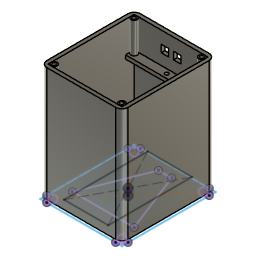
Down_Layer v36 (Autodesk Fusion 360 design; units mm, degrees)
Autodesk Fusion 360 part; units mm, degrees
sketch "Sketch1" plane through (0, 0, 0) normal (0, 0, 1) x (1, 0, 0) in component "Upper Layer"
  line L0 (30, -35) -> (-30, -35)
  line L1 (-30, -35) -> (-30, 35)
  line L2 (-30, 35) -> (30, 35)
  line L3 (30, 35) -> (30, -35)
  line L4 (0, 0) -> (-20, 0) construction
  line L5 (-30, 0) -> (-18, 0) construction
  line L6 (0, -35) -> (0, 35)
  line L7 (-30, -35) -> (0, 0) construction
  line L8 (30, 35) -> (0, 0) construction
  line L9 (-28, 38) -> (28, 38)
  line L10 (33, 33) -> (33, -33)
  line L11 (28, -38) -> (-28, -38)
  line L12 (-33, -33) -> (-33, 33)
  line L13 (-33, 38) -> (33, -38) construction
  line L14 (33, 38) -> (-33, -38) construction
  arc A0 (-33, -33) -> (-28, -38) centre (-28, -33) ccw
  arc A1 (33, 33) -> (28, 38) centre (28, 33) ccw
  arc A2 (28, -38) -> (33, -33) centre (28, -33) ccw
  arc A3 (-28, 38) -> (-33, 33) centre (-28, 33) ccw
  dimension "d1" = 60
  dimension "d2" = 70
  dimension "d27" = 12
  dimension "d33" = 66
  dimension "d34" = 76
  dimension "d110" = 5
  dimension "d111" = 5
  dimension "d112" = 5
  dimension "d113" = 5
  constraint horizontal L0
  constraint perpendicular L0 L1
  constraint parallel L0 L2
  constraint parallel L1 L3
  constraint coincident L4.start L7.end
  constraint horizontal L4
  constraint midpoint L1 L5.start
  constraint perpendicular L1 L5
  constraint midpoint L0 L6.start
  constraint midpoint L2 L6.end
  constraint parallel L7 L8
  constraint horizontal L9
  constraint perpendicular L9 L10
  constraint parallel L9 L11
  constraint parallel L10 L12
  constraint coincident L13 L4.start
  constraint coincident L14 L4.start
  constraint coincident L14.end L11
  constraint coincident L14.end L12
  constraint tangent L11 A0
  constraint tangent L12 A0
  constraint coincident L14.start L10
  constraint coincident L14.start L9
  constraint tangent L10 A1
  constraint tangent L9 A1
  constraint coincident L13.end L10
  constraint coincident L13.end L11
  constraint tangent L10 A2
  constraint tangent L11 A2
  constraint coincident L13.start L9
  constraint coincident L13.start L12
  constraint tangent L9 A3
  constraint tangent L12 A3
  measures "d1" distance of L1.end L2.end
  measures "d2" distance of L0.end L1.end
  measures "d27" distance of L5.start L5.end
  measures "d33" distance of L13.end L14.end
  measures "d34" distance of L14.start L13.end
  measures "d110" radius of A0
  measures "d111" radius of A1
  measures "d112" radius of A2
  measures "d113" radius of A3
extrude "Extrude1" add sketch "Sketch1" along normal blind 5 contours L0 L2 L3 L6 | L0 L1 L2 L6 makes body 1 in component "Upper Layer"
extrude "Extrude8" add sketch "Sketch1" along normal blind 5 contours L0 L2 L3 L6 | L0 L1 L2 L6 | L9 L10 L11 L12 A0 A1 A2 A3 bodies 1 in component "Upper Layer"
sketch "Sketch2" plane through (0, 0, 0) normal (0, 0, 1) x (-1, 0, 0) in component "Upper Layer"
  line L0 (-30, 35) -> (30, 35)
  line L1 (30, 35) -> (30, -35)
  line L2 (30, -35) -> (-30, -35)
  line L3 (-30, -35) -> (-30, 35)
  line L4 (-30, 35) -> (30, -35) construction
  line L5 (30, 35) -> (-30, -35) construction
  line L6 (0, 35) -> (0, -35) construction
  line L7 (2.5, -11) -> (-2.5, -11)
  line L8 (-2.5, -11) -> (-2.5, -20)
  line L9 (-2.5, -20) -> (2.5, -20)
  line L10 (2.5, -20) -> (2.5, -11)
  line L11 (2.5, -11) -> (-2.5, -20) construction
  line L12 (-2.5, -11) -> (2.5, -20) construction
  line L13 (0, -11) -> (0, 9) construction
  line L14 (0, 9) -> (-7.5, 9) construction
  line L15 (-7.5, 9) -> (-15.5, 9)
  line L16 (-15.5, 9) -> (-15.5, 4)
  line L17 (-15.5, 4) -> (-7.5, 4)
  line L18 (-7.5, 4) -> (-7.5, 9)
  line L19 (15.5, 4) -> (7.5, 4)
  line L20 (7.5, 4) -> (7.5, 9)
  line L21 (15.5, 9) -> (15.5, 4)
  line L22 (7.5, 9) -> (15.5, 9)
  line L23 (-5.5, -8) -> (5.5, -8)
  line L24 (5.5, -8) -> (5.5, -23)
  line L25 (5.5, -23) -> (-5.5, -23)
  line L26 (-5.5, -23) -> (-5.5, -8)
  line L27 (-5.5, -8) -> (5.5, -23) construction
  line L28 (5.5, -8) -> (-5.5, -23) construction
  line L29 (-11.5, 9) -> (-11.5, 4) construction
  line L30 (-7.5, 6.5) -> (-15.5, 6.5) construction
  line L31 (-19, 11.5) -> (-4, 11.5)
  line L32 (-4, 11.5) -> (-4, 1.5)
  line L33 (-4, 1.5) -> (-19, 1.5)
  line L34 (-19, 1.5) -> (-19, 11.5)
  line L35 (-19, 11.5) -> (-4, 1.5) construction
  line L36 (-4, 11.5) -> (-19, 1.5) construction
  line L37 (4, 1.5) -> (19, 1.5)
  line L38 (4, 11.5) -> (4, 1.5)
  line L39 (19, 11.5) -> (4, 11.5)
  line L40 (19, 1.5) -> (19, 11.5)
  line L41 (38, 43) -> (-38, 43)
  line L42 (-38, 43) -> (-38, -43)
  line L43 (-38, -43) -> (38, -43)
  line L44 (38, -43) -> (38, 43)
  line L45 (-38, 43) -> (38, 43)
  line L46 (38, 43) -> (38, -43)
  line L47 (38, -43) -> (-38, -43)
  line L48 (-38, -43) -> (-38, 43)
  line L49 (-28, 38) -> (28, 38)
  line L50 (33, 33) -> (33, -33)
  line L51 (28, -38) -> (-28, -38)
  line L52 (-33, -33) -> (-33, 33)
  circle A0 centre (0, -15.5) radius 1.5
  circle A1 centre (-11.5, 6.5) radius 1.5
  circle A2 centre (11.5, 6.5) radius 1.5
  arc A3 (33, 33) -> (28, 38) centre (28, 33) ccw
  arc A4 (-33, -33) -> (-28, -38) centre (-28, -33) ccw
  arc A5 (-28, 38) -> (-33, 33) centre (-28, 33) ccw
  arc A6 (28, -38) -> (33, -33) centre (28, -33) ccw
  line L53 (0, 0) -> (2.5, -15.5) construction
  line L54 (0, 0) -> (0, -30) construction
  line L55 (0, 0) -> (0, 20) construction
  line L56 (0, 20) -> (25, 20)
  line L57 (25, 20) -> (5.2444, -30)
  line L58 (5.2444, -30) -> (-5.5, -30)
  line L59 (0, 20) -> (-25, 20)
  line L60 (-25, 20) -> (-5.5, -30)
  point P0 (0, -15.5)
  point P1 (0, -15.5)
  point P2 (-11.5, 6.5)
  dimension "d7" = 5
  dimension "d8" = 9
  dimension "d9" = 20
  dimension "d10" = 7.5
  dimension "d11" = 8
  dimension "d12" = 5
  dimension "d13" = 11
  dimension "d14" = 15
  dimension "d15" = 15
  dimension "d16" = 10
  dimension "d75" = 3
  dimension "d76" = 3
  dimension "d116" = 25
  dimension "d117" = 25
  constraint horizontal L0
  constraint perpendicular L0 L1
  constraint parallel L0 L2
  constraint parallel L1 L3
  constraint coincident L4 L53.start
  constraint coincident L5 L53.start
  constraint coincident L53.start L54.start
  constraint midpoint L0 L6.start
  constraint midpoint L2 L6.end
  constraint horizontal L7
  constraint perpendicular L7 L8
  constraint parallel L7 L9
  constraint parallel L8 L10
  constraint coincident L11 P1
  constraint coincident L12 P1
  constraint coincident L6 P1
  constraint midpoint L7 L13.start
  constraint perpendicular L7 L13
  constraint perpendicular L13 L14
  constraint horizontal L15
  constraint vertical L16
  constraint horizontal L17
  constraint vertical L18
  constraint symmetric L6 L14.end L20.end
  constraint symmetric L6 L15.end L21.start
  constraint symmetric L6 L16.end L19.start
  constraint symmetric L6 L17.end L19.end
  constraint horizontal L23
  constraint perpendicular L23 L24
  constraint parallel L23 L25
  constraint parallel L24 L26
  constraint coincident L27 P1
  constraint coincident L28 P1
  constraint coincident P1 P0
  constraint midpoint L15 L29.start
  constraint midpoint L17 L29.end
  constraint midpoint L18 L30.start
  constraint midpoint L16 L30.end
  constraint horizontal L31
  constraint perpendicular L31 L32
  constraint parallel L31 L33
  constraint parallel L32 L34
  constraint coincident L35 P2
  constraint coincident L36 P2
  constraint midpoint L29 P2
  constraint symmetric L6 L31.start L39.start
  constraint symmetric L6 L31.end L38.start
  constraint symmetric L6 L32.end L37.start
  constraint symmetric L6 L33.end L37.end
  constraint coincident P2 A1.centre
  constraint symmetric L13 A1 A2
  constraint midpoint L10 L53.end
  constraint coincident L6 L54.end
  constraint perpendicular L25 L54
  constraint coincident L6 L55.end
  constraint perpendicular L39 L55
  constraint perpendicular L6 L56
  constraint perpendicular L26 L58
  constraint perpendicular L6 L59
  measures "d7" distance of L8.end L9.end
  measures "d8" distance of L7.end L8.end
  measures "d9" distance of L13.start L13.end
  measures "d10" distance of L13.end L14.end
  measures "d11" distance of L14.end L15.end
  measures "d12" distance of L14.end L17.end
  measures "d13" distance of L24.end L25.end
  measures "d14" distance of L23.end L24.end
  measures "d15" distance of L32.end L33.end
  measures "d16" distance of L31.end L32.end
  measures "d75" diameter of A0
  measures "d76" diameter of A1
  measures "d116" distance of L55.end L56.end
  measures "d117" distance of L55.end L59.end
extrude "Extrude19" cut sketch "Sketch2" sketch "Sketch1" along normal blind 2 contours L0 L1 L2 L3 | L33 L34 L60 | L37 L40 L57 of sketch 2 bodies 1 in component "Upper Layer"
sketch "Sketch9" plane through (0, 0, 0) normal (0, 0, -1) x (1, 0, 0)
  line L0 (-28, 38) -> (28, 38) construction
  line L1 (33, 33) -> (33, -33) construction
  line L2 (28, -38) -> (-28, -38) construction
  line L3 (-33, -33) -> (-33, 33) construction
  arc A0 (-28, 38) -> (-33, 33) centre (-28, 33) ccw
  arc A1 (28, -38) -> (33, -33) centre (28, -33) ccw
  arc A2 (-33, -33) -> (-28, -38) centre (-28, -33) ccw
  arc A3 (33, 33) -> (28, 38) centre (28, 33) ccw
  line L4 (5.5, -30) -> (25, 20)
  line L5 (25, 20) -> (-25, 20)
  line L6 (-25, 20) -> (-5.2444, -30)
  line L7 (-5.2444, -30) -> (5.5, -30)
extrude "Extrude15" cut sketch "Sketch2" along normal blind 5 contours A0 | A1 | A2 bodies 1 in component "Upper Layer"
extrude "Extrude16" cut sketch "Sketch2" along normal blind 1 contours L7 L8 L9 L10 | L15 L16 L17 L18 | L19 L20 L21 L22 bodies 1 in component "Upper Layer"
sketch "Sketch6" plane through (0, 0, 5) normal (0, 0, 1) x (-1, 0, 0) in component "Upper Layer"
  line L0 (28, 38) -> (-28, 38)
  line L1 (-33, 33) -> (-33, -33)
  line L2 (-28, -38) -> (28, -38)
  line L3 (33, -33) -> (33, 33)
  line L4 (30, 35) -> (30, -35)
  line L5 (30, -35) -> (-30, -35)
  line L6 (-30, -35) -> (-30, 35)
  line L7 (-30, 35) -> (30, 35)
  line L8 (-28, 38) -> (28, 38)
  line L9 (-33, -33) -> (-33, 33)
  line L10 (28, -38) -> (-28, -38)
  line L11 (33, 33) -> (33, -33)
  circle A0 centre (0, -15.5) radius 1.5
  circle A1 centre (-11.5, 6.5) radius 1.5
  circle A2 centre (11.5, 6.5) radius 1.5
  arc A3 (33, 33) -> (28, 38) centre (28, 33) ccw
  arc A4 (-33, -33) -> (-28, -38) centre (-28, -33) ccw
  arc A5 (28, -38) -> (33, -33) centre (28, -33) ccw
  arc A6 (-28, 38) -> (-33, 33) centre (-28, 33) ccw
ref_plane "WorkPlane1" through (0, 0, 25) normal (0, 0, 1) x (1, 0, 0)
extrude "Extrude9" add sketch "Sketch6" along normal blind 90 contours L0 L1 L2 L3 L8 L9 L10 L11 A3 A4 A5 A6 bodies 1 in component "Upper Layer"
sketch "Sketch5" plane through (0, 35, 0) normal (0, -1, 0) x (1, 0, 0)
  line L0 (-30, 5) -> (30, 5)
  line L1 (30, 5) -> (30, 95)
  line L2 (30, 95) -> (-30, 95)
  line L3 (-30, 95) -> (-30, 5)
  line L4 (-30, 95) -> (-30, 73) construction
  line L5 (-30, 73) -> (-30, 70) construction
  line L6 (-30, 70) -> (30, 70)
  line L7 (30, 70) -> (30, 67)
  line L8 (30, 67) -> (-30, 67)
  line L9 (-30, 67) -> (-30, 70)
  dimension "d58" = 22
  dimension "d59" = 3
  dimension "d60" = 3
  constraint coincident L2.end L3.start
  constraint perpendicular L2 L4
  constraint parallel L3 L5
  constraint horizontal L6
  constraint vertical L7
  constraint horizontal L8
  constraint vertical L9
  measures "d58" distance of L2.end L4.end
  measures "d59" distance of L4.end L5.end
  measures "d60" distance of L5.end L8.end
sketch "Sketch6 (2)" plane through (0, -35, 0) normal (0, 1, 0) x (-1, 0, 0)
  line L0 (-30, 5) -> (30, 5)
  line L1 (30, 5) -> (30, 95)
  line L2 (30, 95) -> (-30, 95)
  line L3 (-30, 95) -> (-30, 5)
  line L4 (-30, 95) -> (-30, 73) construction
  line L5 (-30, 73) -> (-30, 70) construction
  line L6 (-30, 70) -> (30, 70)
  line L7 (30, 70) -> (30, 67)
  line L8 (30, 67) -> (-30, 67)
  line L9 (-30, 67) -> (-30, 70)
  dimension "d61" = 22
  dimension "d62" = 3
  dimension "d63" = 3
  constraint coincident L2.end L3.start
  constraint perpendicular L2 L4
  constraint parallel L3 L5
  constraint horizontal L6
  constraint vertical L7
  constraint horizontal L8
  constraint vertical L9
  measures "d61" distance of L2.end L4.end
  measures "d62" distance of L4.end L5.end
  measures "d63" distance of L5.end L8.end
extrude "Extrude12" add sketch "Sketch6 (2)" along normal blind 7 contours L1 L3 L6 L7 L8 L9 bodies 1 in component "Upper Layer"
extrude "Extrude13" add sketch "Sketch5" along normal blind 7 contours L1 L3 L6 L7 L8 L9 bodies 1 in component "Upper Layer"
sketch "Sketch7" plane through (0, 0, 70) normal (0, 0, 1) x (-1, 0, 0)
  line L0 (30, 35) -> (-30, 35)
  line L1 (-30, 35) -> (-30, 28)
  line L2 (-30, 28) -> (30, 28)
  line L3 (30, 28) -> (30, 35)
  line L4 (30, 31.5) -> (-30, 31.5)
  line L5 (0, 35) -> (0, 28)
  circle A0 centre (0, 31.5) radius 1.5
  dimension "d92" = 3
  constraint midpoint L3 L4.start
  constraint midpoint L1 L4.end
  constraint midpoint L0 L5.start
  constraint midpoint L2 L5.end
  constraint midpoint L4 A0.centre
  measures "d92" diameter of A0
sketch "Sketch8" plane through (0, 0, 70) normal (0, 0, 1) x (-1, 0, 0)
  line L0 (-30, -35) -> (30, -35)
  line L1 (30, -35) -> (30, -28)
  line L2 (30, -28) -> (-30, -28)
  line L3 (-30, -28) -> (-30, -35)
  line L4 (30, -31.5) -> (-30, -31.5)
  line L5 (0, -28) -> (0, -35)
  circle A0 centre (0, -31.5) radius 1.5
  dimension "d93" = 3
  constraint midpoint L1 L4.start
  constraint midpoint L3 L4.end
  constraint midpoint L2 L5.start
  constraint midpoint L0 L5.end
  constraint midpoint L4 A0.centre
  measures "d93" diameter of A0
sketch "Sketch10" plane through (0, 0, 25) normal (0, 0, 1) x (1, 0, 0)
  line L0 (-30, -35) -> (-12, -35)
  line L1 (-30, -35) -> (-30, -17)
  line L2 (-30, -17) -> (-12, -35)
  line L3 (30, 35) -> (12, 35)
  line L4 (30, 35) -> (30, 17)
  line L5 (30, 17) -> (12, 35)
  line L6 (30, -35) -> (12, -35)
  line L7 (30, -35) -> (30, -17)
  line L8 (12, -35) -> (30, -17)
  line L9 (-30, 35) -> (-30, 17)
  line L10 (-30, 35) -> (-12, 35)
  line L11 (-12, 35) -> (-30, 17)
  dimension "d82" = 18
  dimension "d83" = 18
  dimension "d84" = 18
  dimension "d85" = 18
  dimension "d86" = 18
  dimension "d89" = 18
  dimension "d90" = 18
  dimension "d91" = 18
  constraint horizontal L0
  constraint perpendicular L0 L1
  constraint horizontal L3
  constraint perpendicular L3 L4
  constraint perpendicular L4 L6
  constraint perpendicular L6 L7
  constraint perpendicular L6 L9
  constraint perpendicular L9 L10
  measures "d82" distance of L0.start L0.end
  measures "d83" distance of L3.start L3.end
  measures "d84" distance of L3.start L4.end
  measures "d85" distance of L6.start L6.end
  measures "d86" distance of L9.start L9.end
  measures "d89" distance of L9.start L10.end
  measures "d90" distance of L6.start L7.end
  measures "d91" distance of L0.start L1.end
extrude "Extrude17" add sketch "Sketch10" against normal blind 2 bodies 1 in component "Upper Layer"
sketch "Sketch4" plane through (0, 38, 0) normal (0, 1, 0) x (-1, 0, 0)
  line L0 (28, 95) -> (-28, 95)
  line L1 (33, 79) -> (8, 79) construction
  line L2 (8, 79) -> (2, 79)
  line L3 (2, 79) -> (2, 85)
  line L4 (2, 85) -> (8, 85)
  line L5 (8, 85) -> (8, 79)
  line L6 (0, 95) -> (0, 0)
  line L7 (-8, 85) -> (-8, 79)
  line L8 (-8, 79) -> (-2, 79)
  line L9 (-2, 85) -> (-8, 85)
  line L10 (-2, 79) -> (-2, 85)
  line L11 (28, 2) -> (28, 95)
  line L12 (-28, 95) -> (-28, 2)
  line L13 (-28, 2) -> (28, 2)
  dimension "d53" = 25
  dimension "d54" = 6
  dimension "d55" = 6
  dimension "d94" = 10
  constraint horizontal L2
  constraint vertical L3
  constraint horizontal L4
  constraint vertical L5
  constraint midpoint L0 L6.start
  constraint coincident L6.end origin
  constraint symmetric L1.end L6 L7.end
  constraint symmetric L2.end L6 L8.end
  constraint symmetric L3.end L6 L9.start
  constraint symmetric L4.end L6 L7.start
  measures "d53" distance of L1.start L1.end
  measures "d54" distance of L1.end L2.end
  measures "d55" distance of L1.end L4.end
  measures "d94" distance of L0 L4.end
extrude "Extrude11" cut sketch "Sketch4" against normal blind 8 contours L2 L3 L4 L5 | L7 L8 L9 L10 bodies 1 in component "Upper Layer"
sketch "Sketch12" plane through (0, 0, 70) normal (0, 0, 1) x (-1, 0, 0)
  line L0 (30, 35) -> (-30, 35)
  line L1 (-30, 35) -> (-30, 28)
  line L2 (-30, 28) -> (30, 28)
  line L3 (30, 28) -> (30, 35)
  line L4 (0, 28) -> (0, 35)
  circle A0 centre (0, 31.5) radius 1.5
  line L5 (-30, 35) -> (-27.5, 35) construction
  line L6 (-27.5, 35) -> (-27.5, 32.5) construction
  line L7 (-27.5, 32.5) -> (-30, 32.5) construction
  line L8 (-30, 32.5) -> (-30, 35) construction
  circle A1 centre (-27.5, 32.5) radius 2.5
  circle A2 centre (-27.5, 32.5) radius 1.5
  circle A3 centre (27.5, 32.5) radius 2.5
  circle A4 centre (27.5, 32.5) radius 1.5
  dimension "d95" = 3
  dimension "d99" = 2.5
  dimension "d100" = 2.5
  dimension "d101" = 3
  constraint midpoint L2 L4.start
  constraint midpoint L0 L4.end
  constraint midpoint L4 A0.centre
  constraint horizontal L5
  constraint vertical L6
  constraint horizontal L7
  constraint vertical L8
  constraint coincident L0.end L1.start
  constraint coincident L5.end A1
  constraint coincident L7.end A1
  constraint tangent L8 A1
  constraint concentric A1 A2
  constraint symmetric L4 A1 A3
  constraint symmetric L4 A2 A4
  measures "d95" diameter of A0
  measures "d99" distance of L0.end L5.end
  measures "d100" distance of L0.end L7.end
  measures "d101" diameter of A2
sketch "Sketch13" plane through (0, 0, 70) normal (0, 0, 1) x (-1, 0, 0)
  line L0 (-30, -35) -> (30, -35)
  line L1 (30, -35) -> (30, -28)
  line L2 (30, -28) -> (-30, -28)
  line L3 (-30, -28) -> (-30, -35)
  line L4 (0, -35) -> (0, -28)
  circle A0 centre (0, -31.5) radius 1.5
  line L5 (-30, -35) -> (-27.5, -35) construction
  line L6 (-27.5, -35) -> (-27.5, -32.5) construction
  line L7 (-27.5, -32.5) -> (-30, -32.5) construction
  line L8 (-30, -32.5) -> (-30, -35) construction
  circle A1 centre (-27.5, -32.5) radius 2.5
  circle A2 centre (-27.5, -32.5) radius 1.5
  circle A3 centre (27.5, -32.5) radius 1.5
  circle A4 centre (27.5, -32.5) radius 2.5
  dimension "d96" = 3
  dimension "d102" = 2.5
  dimension "d103" = 2.5
  dimension "d104" = 3
  dimension "d122" = 31.5
  dimension "d123" = 42.5735
  constraint midpoint L0 L4.start
  constraint midpoint L2 L4.end
  constraint midpoint L4 A0.centre
  constraint horizontal L5
  constraint vertical L6
  constraint horizontal L7
  constraint vertical L8
  constraint coincident L0.start L3.end
  constraint coincident L5.end A1
  constraint coincident L7.end A1
  constraint tangent L5 A1
  constraint concentric A1 A2
  constraint symmetric L4 A1 A4
  constraint symmetric L4 A2 A3
  measures "d96" diameter of A0
  measures "d102" distance of L0.start L5.end
  measures "d103" distance of L0.start L7.end
  measures "d104" diameter of A2
  measures "d122" distance of origin A0.centre
  measures "d123" distance of origin A3.centre
extrude "Extrude18" cut sketch "Sketch13" sketch "Sketch12" against normal blind 3 contours L4 A0 | L4 A0 of sketch 2 contours L4 A0 | L4 A0 bodies 1 in component "Upper Layer"
ref_plane "WorkPlane2" through (0, 0, 95) normal (0, 0, 1) x (-1, 0, 0)
extrude "Extrude1'" add sketch "Sketch13" along normal up to surface (25 mm away) separate body contours A1 | A4 makes body 2 at (29.8037, 33.4711, 86.6667) makes body 3 at (-25.1963, 33.4711, 86.6667)
extrude "Extrude2" add sketch "Sketch12" along normal up to surface (25 mm away) separate body contours A3 | A1 makes body 4 at (29.4151, -34.107, 86.6667) makes body 5 at (-25.3044, -33.6956, 78.3333)
sketch "Sketch1 (2)" plane through (0, 0, 0) normal (0, 0, 1) x (1, 0, 0)
  line L0 (33.1828, -38.1163) -> (-33.1828, -38.1163)
  line L1 (-33.1828, -38.1163) -> (-33.1828, 38.1163)
  line L2 (-33.1828, 38.1163) -> (33.1828, 38.1163)
  line L3 (33.1828, 38.1163) -> (33.1828, -38.1163)
  line L4 (33.1828, -38.1163) -> (-33.1828, 38.1163) construction
  line L5 (-33.1828, -38.1163) -> (33.1828, 38.1163) construction
  constraint horizontal L0
  constraint perpendicular L0 L1
  constraint parallel L0 L2
  constraint parallel L1 L3
  constraint coincident L4 origin
  constraint coincident L5 origin
sketch "Sketch14" plane through (0, 0, 5) normal (0, 0, 1) x (-1, 0, 0)
  line L0 (-30, -35) -> (30, -35)
  line L1 (30, -35) -> (30, 35)
  line L2 (30, 35) -> (-30, 35)
  line L3 (-30, 35) -> (-30, -35)
  circle A0 centre (0, -15.5) radius 1.5
  circle A1 centre (-11.5, 6.5) radius 1.5
  circle A2 centre (11.5, 6.5) radius 1.5
  line L4 (18, -34) -> (-18, -34)
  line L5 (-18, -34) -> (-18, 34)
  line L6 (-18, 34) -> (18, 34)
  line L7 (18, 34) -> (18, -34)
  line L8 (18, -34) -> (-18, 34) construction
  line L9 (-18, -34) -> (18, 34) construction
  dimension "d120" = 36
  dimension "d121" = 68
  constraint horizontal L4
  constraint perpendicular L4 L5
  constraint parallel L4 L6
  constraint parallel L5 L7
  constraint coincident L8 origin
  constraint coincident L9 origin
  measures "d120" distance of L4.start L4.end
  measures "d121" distance of L4.end L5.end
imported_body "Base Feature1" makes body 6 in component "97710A134_18-8 Stainless Steel Narrow Cheese Head Slotted Screws"
component "Upper Layer" placed x (1, 0, 0) y (0, 1, 0) z (0, 0, 1) at (0, 0, 0)
equation "d10 = ( 15 / 2 ) * 1 mm"
